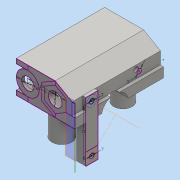
# Autodesk Inventor part: XMountL
Saved by Autodesk Inventor 2016 (Build 200138000, 138)
## iProperties
Created: 2016-08-28
Part Number: XMountL
Material: Generic
Document SubType Name: Modeling
Designer: Sam
Density: 1 g/cm^3
Appearance: Default
Author: Sam
Autodesk Inventor part; units mm, degrees
ref_plane "YZ Plane" through (0, 0, 0) normal (1, 0, 0) x (0, 1, 0)
ref_plane "XZ Plane" through (0, 0, 0) normal (0, 1, 0) x (-1, 0, 0)
ref_plane "XY Plane" through (0, 0, 0) normal (0, 0, 1) x (1, 0, 0)
sketch "Sketch1" plane through (0, 0, 0) normal (1, 0, 0) x (0, 1, 0)
  circle A0 centre (0, 0) radius 1.5
  circle A1 centre (0, -31) radius 1.5
  circle A2 centre (0, 0) radius 3.5 construction
  circle A3 centre (0, -31) radius 3.5 construction
  line L0 (4, 4) -> (-4, 4)
  line L1 (-4, 4) -> (-4, -35)
  line L2 (-4, -35) -> (4, -35)
  line L3 (4, -35) -> (4, 4)
  line L4 (-4, -35) -> (4, -35)
  line L5 (-4, -27) -> (-4, -35)
  line L6 (31, -31) -> (0, 0) construction
  line L7 (0, -31) -> (15.5, -15.5) construction
  circle A4 centre (31, 1.5) radius 1.5
  line L8 (4, -27) -> (-4, -27)
  dimension "d0" = 3
  dimension "d1" = 3
  dimension "d3" = 31
  dimension "d6" = 7
  dimension "d7" = 7
  dimension "d64" = 3
  constraints: 18 end point, 5 centre point, 3 coincident, 3 parallel, 2 horizontal, 1 midpoint, 1 perpendicular, 1 point on line
  measures "d0" diameter of A0
  measures "d1" diameter of A1
  measures "d3" distance of A1.centre point (0, 0)
  measures "d6" diameter of A2
  measures "d7" diameter of A3
  measures "d64" diameter of A4
extrude "Extrusion1" add sketch "Sketch1" against normal blind 6 contours L3 L8 L1 L0 | L3 L2 L1 L8
ref_plane "Work Plane6" through (0, -11, 4) normal (0, 1, 0) x (1, 0, 0)
sketch "Sketch2" plane through (0, -11, 4) normal (0, 1, 0) x (1, 0, 0)
  line L0 (-6.023191, 2.500092) -> (-6.023191, 5.500092) construction
  line L1 (-6.023191, 4.000092) -> (-13.023191, 4.000092) construction
  line L2 (-6.041071, 8.03122) -> (-6.041071, 4.000092)
  line L3 (-6.041071, -0.031037) -> (-13.023191, -4.062166)
  line L4 (-13.023191, -4.062166) -> (-20.005311, -0.031037)
  line L5 (-20.005311, -0.031037) -> (-20.005311, 8.03122)
  line L6 (-20.005311, 8.03122) -> (-13.023191, 12.062349)
  line L7 (-13.023191, 12.062349) -> (-6.041071, 8.03122)
  line L8 (-22.03646, 9.203905) -> (-22.03646, -1.203722)
  line L9 (-22.03646, -1.203722) -> (-13.023191, -6.407535)
  line L10 (-13.023191, 14.407718) -> (-22.03646, 9.203905)
  line L11 (-13.023191, 4.000092) -> (-31.023191, 4.000092) construction
  circle A0 centre (-31.023191, 4.000092) radius 7.5
  line L12 (-13.023191, -6.407535) -> (-30.97685, -6.407535)
  line L13 (-30.97685, -6.407535) -> (-30.97685, -3.499765)
  line L14 (-30.97685, 11.499948) -> (-30.97685, 14.407718)
  line L15 (-30.97685, 14.407718) -> (-13.023191, 14.407718)
  circle A1 centre (-13.023191, 4.000092) radius 4.5
  line L16 (-30.97685, 11.499988) -> (-30.97685, 14.407718)
  line L17 (-30.97685, -3.500012) -> (-30.97685, -6.407535)
  line L18 (-13.023191, -4.062166) -> (-13.023191, -6.407535)
  line L19 (-13.023191, 12.062349) -> (-13.023191, 14.407718)
  line L20 (-6.041071, 4.000092) -> (-6.041071, -0.031037)
  line L21 (-13.023191, 14.407718) -> (0, 14.407718)
  line L22 (0, 39) -> (0, 0)
  line L23 (0, 14.407718) -> (0, 8.03122)
  line L24 (0, 8.03122) -> (-6.041071, 8.03122)
  line L25 (0, 0) -> (-6, 0)
  line L26 (-13.023191, -6.407535) -> (-2, 0)
  line L27 (-2, 0) -> (-2, 8.03122)
  line L28 (-2, 0) -> (0, 0)
  line L29 (0, 8.03122) -> (0, 0)
  circle A2 centre (-31.023191, 4.000092) radius 4
  line L30 (-30.97685, -3.500012) -> (-38.523191, -3.500012)
  line L31 (-38.523191, -3.500012) -> (-38.523191, -6.407535)
  line L32 (-38.523191, -6.407535) -> (-30.97685, -6.407535)
  line L33 (-30.97685, -6.407535) -> (-30.97685, -3.500012)
  line L34 (-30.97685, 14.407718) -> (-38.523191, 14.407718)
  line L35 (-38.523191, 14.407718) -> (-38.523191, 11.499988)
  line L36 (-38.523191, 11.499988) -> (-30.97685, 11.499988)
  line L37 (-30.97685, 11.499988) -> (-30.97685, 14.407718)
  point P0 (0, 31)
  dimension "d11" = 7
  dimension "d12" = 18
  dimension "d13" = 15
  dimension "d16" = 9
  dimension "d70" = 8
  constraints: 72 end point, 7 perpendicular, 6 point on line, 5 horizontal, 4 coincident, 4 parallel, 3 centre point, 2 collinear, 2 point on circle, 1 midpoint, 1 vertical, 14 other
  measures "d11" distance of L1.start L1.end
  measures "d12" distance of L11.start L11.end
  measures "d13" diameter of A0
  measures "d16" diameter of A1
  measures "d70" diameter of A2
extrude "Extrusion6" add sketch "Sketch2" along normal blind 5 contours L2 L20 L3 L4 L5 L6 L7
extrude "Extrusion5" add sketch "Sketch2" along normal blind 58 contours L24 L27 L26 L18 L3 L20 L2 | L7 L19 L21 L22 L24 | L6 L5 L4 L18 L9 L8 L10 L19 | L10 L8 L9 L12 L13 A0 L14 L15 | L14 L36 L35 L34 | L32 L31 L30 L13
sketch "Sketch6" plane through (0, 0, 0) normal (1, 0, 0) x (0, 0, -1)
  circle A0 centre (0, 0) radius 1.5 construction
  line L0 (25.11, 30.435307) -> (0, 0) construction
  circle A1 centre (31, 0) radius 1.5 construction
  line L1 (31, 0) -> (12.555, 15.217653) construction
  circle A2 centre (12.555, 15.217653) radius 9
  dimension "d51" = 18
  constraints: 4 end point, 1 centre point, 1 coincident, 1 midpoint, 1 perpendicular
  measures "d51" diameter of A2
sketch "Sketch7" plane through (0, -11, -10.407718) normal (0, 0, -1) x (-1, 0, 0)
  line L0 (0, 46) -> (0, 15) construction
  line L1 (0, 26.436517) -> (15, 26.436517) construction
  line L2 (15, 26.436517) -> (15, 6.436517) construction
  line L3 (15, 26.436517) -> (15, 46.436517) construction
  circle A0 centre (15, 6.436517) radius 4
  circle A1 centre (15, 46.436517) radius 4
  circle A2 centre (15, 46.436517) radius 6.068392
  circle A3 centre (15, 6.436517) radius 6.52468
  point P0 (0, 11)
  dimension "d52" = 20
  dimension "d53" = 20
  dimension "d54" = 8
  dimension "d55" = 8
  dimension "d60" = 2.06839
  dimension "d61" = 2.52468
  constraints: 6 end point, 4 centre point, 2 coincident, 2 vertical, 1 horizontal, 1 point on line
  measures "d52" distance of L1.end L2.end
  measures "d53" distance of L1.end L3.end
  measures "d54" diameter of A0
  measures "d55" diameter of A1
  measures "d60" radial gap between concentric circles of A1 A2
  measures "d61" radial gap between concentric circles of A0 A3
extrude "Extrusion8" add sketch "Sketch7" along normal blind 15
extrude "Extrusion9" cut sketch "Sketch6" against normal through all
extrude "Extrusion10" cut sketch "Sketch1" against normal through all contours A0
extrude "Extrusion11" cut sketch "Sketch1" against normal through all contours A4
sketch "Sketch8" plane through (0, 47, 4) normal (0, 1, 0) x (1, 0, 0)
  circle A0 centre (-31, 4) radius 5
  circle A1 centre (-31, 4) radius 7.5
  point P0 (0, 4)
  dimension "d67" = 15
  constraints: 2 centre point, 1 coincident
  measures "d67" diameter of A1
extrude "Extrusion12" add sketch "Sketch8" against normal blind 2
sketch "Sketch2 outline for Extrusion13" plane through (0, -11, 4) normal (0, 1, 0) x (1, 0, 0)
  arc A0 (-30.97685, 11.499948) -> (-30.97685, -3.499765) centre (-31.023191, 4.000092) ccw
  arc A1 (-30.97685, -3.499765) -> (-30.97685, 11.499948) centre (-31.023191, 4.000092) ccw
  circle A2 centre (-31.023191, 4.000092) radius 4
extrude "Extrusion13" add sketch "Sketch2 outline for Extrusion13" along normal blind 2
sketch "Sketch9" plane through (0, 47, 4) normal (0, 1, 0) x (1, 0, 0)
  point P0 (0, 4)
body "Solid1"
